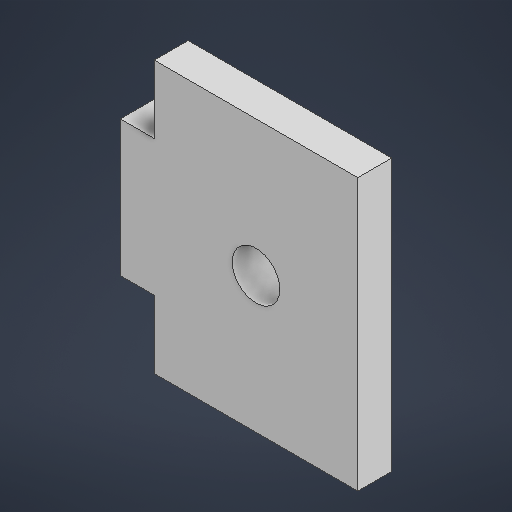
# Autodesk Inventor part: Part8
Saved by Autodesk Inventor 2026.2 (Build 302298000, 298)
## iProperties
Created: 2026-04-17
Part Number: Part8
Material: Generic
Document SubType Name: Modeling
Designer: danda
Density: 1 g/cm^3
Appearance: Default
Author: danda
Autodesk Inventor part; units mm, degrees
ref_plane "YZ Plane" through (0, 0, 0) normal (1, 0, 0) x (0, 1, 0)
ref_plane "XZ Plane" through (0, 0, 0) normal (0, 1, 0) x (-1, 0, 0)
ref_plane "XY Plane" through (0, 0, 0) normal (0, 0, 1) x (1, 0, 0)
sketch "Sketch1" plane through (0, 0, 0) normal (0, 0, 1) x (1, 0, 0)
  line L0 (9.7809, 25.2857) -> (14.7809, 25.2857)
  line L1 (14.7809, 25.2857) -> (14.7809, 5.2857)
  line L2 (14.7809, 5.2857) -> (9.7809, 5.2857)
  line L3 (9.7809, 5.2857) -> (9.7809, 25.2857)
  line L4 (14.7809, 35.2857) -> (44.7809, 35.2857)
  line L5 (44.7809, 35.2857) -> (44.7809, -4.7143)
  line L6 (44.7809, -4.7143) -> (14.7809, -4.7143)
  line L7 (14.7809, -4.7143) -> (14.7809, 35.2857)
  circle A0 centre (29.7809, 15.2857) radius 3.5
  point P0 (0, 0)
  point P1 (12.2809, 25.2857)
  dimension "d0" = 5
  dimension "d1" = 20
  dimension "d2" = 30
  dimension "d3" = 40
  dimension "d4" = 10
  dimension "d7" = 7
  constraints: 16 end point, 4 parallel, 2 horizontal, 2 perpendicular, 1 centre point, 1 midpoint, 1 point on line
  measures "d0" distance of L1.end L2.end
  measures "d1" distance of L0.end L1.end
  measures "d2" distance of L5.end L6.end
  measures "d3" distance of L4.end L5.end
  measures "d4" vertical distance of point (12.281, 25.286) L4.start
  measures "d7" diameter of A0
extrude "Extrusion1" add sketch "Sketch1" along normal blind 5 contours L0 L1 L2 L3 | L7 L4 L5 L6 L1 | A0
extrude "Extrusion2" cut sketch "Sketch1" along normal blind 5 contours A0
body "Solid1"
